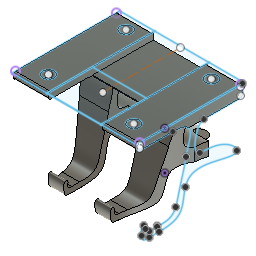
back-long (Autodesk Fusion 360 design; units mm, degrees)
Autodesk Fusion 360 part; units mm, degrees
sketch "Skizze1" plane through (0, 0, 0) normal (1, 0, 0) x (0, 1, 0)
  line L0 (-6.5006, 9.9908) -> (19.5, 9.9908)
  line L1 (20, 9.4908) -> (20, 8.1908)
  line L2 (-7.0006, 8.7446) -> (-7.0006, 9.4908)
  line L3 (-6.5006, 8.2446) -> (2, 8.2446)
  line L4 (10.0033, 7.0396) -> (19.4979, 7)
  line L5 (20, 7.5) -> (20, 8.1908)
  arc A0 (-6.5006, 9.9908) -> (-7.0006, 9.4908) centre (-6.5006, 9.4908) ccw
  arc A1 (-7.0006, 8.7446) -> (-6.5006, 8.2446) centre (-6.5006, 8.7446) ccw
  arc A2 (20, 9.4908) -> (19.5, 9.9908) centre (19.5, 9.4908) ccw
  arc A3 (19.4979, 7) -> (20, 7.5) centre (19.5, 7.5) ccw
  line L6 (-2, -11) -> (-2, -10.8002)
  spline S0 degree 5 poles (5.4564, 0.8875) (5.3855, 0.5136) (5.2329, -0.2254) (4.971, -1.3069) (4.5724, -2.7088) (4.0604, -4.4438) (3.5996, -6.1979) (3.1763, -7.9202) (2.7188, -9.497) (1.8719, -10.5223) (0.6223, -10.9522) (-0.5021, -11.0045) (-1.2907, -11.0008) (-1.7711, -11) (-2, -11) knots 0 0 0 0 0 0 0.1 0.2 0.3 0.4 0.5 0.6 0.7 0.8 0.9 1 1 1 1 1 1
  line L7 (-1, -11) -> (-3, -11)
  line L8 (5.6749, 2.0411) -> (5.2379, -0.266)
  spline S1 degree 5 poles (2, 8.2446) (2.8977, 8.2305) (4.4395, 8.0987) (5.9921, 7.5904) (6.778, 6.3951) (6.5221, 4.4543) (5.9835, 2.8697) (5.6586, 1.8097) (5.5121, 1.1818) (5.4564, 0.8875) knots 0 0 0 0 0 0 0.2 0.4 0.6 0.8 1 1 1 1 1 1
  line L9 (1.6903, 8.2495) -> (2.3097, 8.2397)
  line L10 (3.1911, -8.044) -> (2.3942, -9.956)
  line L11 (-1.4778, -12.3862) -> (-4, -12.3862)
  line L12 (-2, -11) -> (-4, -11)
  spline S2 degree 5 poles (-4, -12.3862) (-4.1637, -12.3825) (-4.4687, -12.3751) (-4.8588, -12.364) (-5.2518, -12.336) (-5.5755, -12.2143) (-5.7856, -11.9369) (-5.929, -11.4713) (-6.0363, -10.8339) (-6.0945, -10.1719) (-6.0772, -9.6063) (-5.9643, -9.2033) (-5.7546, -8.9907) (-5.4704, -8.9625) (-5.1907, -9.0678) (-5.0099, -9.2564) (-4.9465, -9.5244) (-4.9801, -9.8639) (-5.0384, -10.2433) (-5.0135, -10.5787) (-4.8541, -10.8326) (-4.5967, -10.9534) (-4.3278, -10.9955) (-4.1149, -11.0021) (-4, -11) knots 0 0 0 0 0 0 0.05 0.1 0.15 0.2 0.25 0.3 0.35 0.4 0.45 0.5 0.55 0.6 0.65 0.7 0.75 0.8 0.85 0.9 0.95 1 1 1 1 1 1
  line L13 (-3.0067, -12.4087) -> (-4.9933, -12.3637)
  line L14 (-5.782, -8.9412) -> (-5.1061, -9.0588)
  line L15 (-4.9315, -9.3688) -> (-5.0685, -10.6312)
  spline S3 degree 5 poles (-1.4778, -12.3862) (-0.8155, -12.3824) (0.4148, -12.3369) (1.9774, -12.1542) (3.4957, -11.6229) (4.4942, -10.2077) (4.8939, -8.0285) (5.1389, -5.3096) (6.4672, -3.4256) (9.3305, -3.0948) (13.0319, -3.8228) (16.5001, -4.7482) (18.6604, -4.9823) (18.8379, -4.0148) (17.5015, -2.4676) (15.2406, -1.0314) (12.6174, -0.2148) (10.1815, -0.0512) (8.3782, -0.213) (7.5748, 1.0515) (7.7465, 3.7291) (8.456, 5.8911) (9.1756, 6.8309) (9.7171, 7.0396) (10.0033, 7.0396) knots 0 0 0 0 0 0 0.05 0.1 0.15 0.2 0.25 0.3 0.35 0.4 0.45 0.5 0.55 0.6 0.65 0.7 0.75 0.8 0.85 0.9 0.95 1 1 1 1 1 1
  line L16 (-5.5492, -12.4096) -> (2.5937, -12.3628)
  line L17 (18.4871, -5.1308) -> (18.6154, -3.4332)
  line L18 (4.5138, -8.2258) -> (6.0937, -3.3604)
  line L19 (8.3709, 7.0396) -> (11.6358, 7.0396)
  line L20 (10.8658, -0.437) -> (7.1342, 0.437)
  line L21 (-5.8826, -11.7779) -> (-6.1174, -10.2221)
  point P0 (20, 9.9908)
  point P1 (2.7926, -9)
  point P2 (-6, -11)
  point P3 (-5.444, -9)
  point P4 (-5, -10)
  point P5 (5.3038, -5.7931)
  point P6 (18.5512, -4.282)
  point P7 (9, 0)
  dimension "d12" = 0.5
  constraint horizontal L0
  constraint perpendicular L0 L1
  constraint perpendicular L0 L2
  constraint perpendicular L2 L3
  constraint tangent L0 A0
  constraint tangent L2 A0
  constraint tangent L2 A1
  constraint tangent L3 A1
  constraint equal A0 A1
  constraint coincident P0 L0
  constraint coincident P0 L1
  constraint tangent L0 A2
  constraint tangent L1 A2
  constraint equal A0 A2
  constraint tangent L4 A3
  constraint tangent L5 A3
  constraint equal A0 A3
  constraint midpoint L8 S0.start
  constraint midpoint L3.end L9
  constraint midpoint P1 L10
  constraint midpoint L7 L6.start
  constraint midpoint L11.end L13
  constraint midpoint P3 L14
  constraint midpoint P4 L15
  constraint midpoint L11.start L16
  constraint midpoint P6 L17
  constraint midpoint P5 L18
  constraint midpoint L4.start L19
  constraint parallel L0 L19
  constraint midpoint P7 L20
  constraint midpoint P2 L21
  measures "d12" radius of A0
extrude "Extrusion1" add sketch "Skizze1" against normal blind 32 contours L0 L1 L2 L3 L4 L5 A0 A1 A2 A3 S0 L7 S1 L11 L12 S2 S3 makes body 1
sketch "Skizze2" plane through (0, 0, 9.9908) normal (0, 0, 1) x (-1, 0, 0)
  line L0 (0, 6.5006) -> (0, -19.5)
  line L1 (32, -19.5) -> (32, 6.5006)
  line L2 (16, 0) -> (16, -20) construction
  line L3 (0, -20.4) -> (0, 0)
  circle A0 centre (27, -17) radius 1.5
  circle A1 centre (5, -17) radius 1.5
  line L4 (32, -20.3851) -> (23, -20.3851)
  line L5 (23, -20.3851) -> (23, 7.4)
  line L6 (23, 7.4) -> (32, 7.4)
  line L7 (32, 7.4) -> (32, -20.3851)
  line L8 (0, -20.4) -> (9, -20.4)
  line L9 (9, -20.4) -> (9, 7.4031)
  line L10 (9, 7.4031) -> (0, 7.4031)
  line L11 (0, 7.4031) -> (0, -20.4)
  line L12 (23, -20.3851) -> (9, -20.3851)
  line L13 (9, -20.3851) -> (9, 7.4031)
  line L14 (9, 7.4031) -> (23, 7.4031)
  line L15 (23, 7.4031) -> (23, -20.3851)
  circle A2 centre (27, 3) radius 1.5
  circle A3 centre (5, 3) radius 1.5
  line L16 (23, 7.4) -> (9, 7.4)
  line L17 (9, 7.4) -> (9, -4.3434)
  line L18 (9, -4.3434) -> (23, -4.3434)
  line L19 (23, -4.3434) -> (23, 7.4)
  dimension "d6" = 3
  dimension "d7" = 3
  dimension "d23" = 3
  dimension "d24" = 3
  constraint coincident L3.end origin
  constraint horizontal L4
  constraint vertical L5
  constraint horizontal L6
  constraint vertical L7
  constraint horizontal L8
  constraint horizontal L10
  constraint vertical L11
  constraint horizontal L12
  constraint vertical L13
  constraint horizontal L14
  constraint vertical L15
  constraint horizontal L16
  constraint vertical L17
  constraint horizontal L18
  constraint vertical L19
  constraint coincident L9 L17.end
  constraint coincident L13 L17.end
  measures "d6" diameter of A0
  measures "d7" diameter of A1
  measures "d23" diameter of A2
  measures "d24" diameter of A3
extrude "Extrusion3" cut sketch "Skizze2" against normal blind 3 contours A0 | A1 bodies 1
sketch "Skizze3" plane through (0, 0, 0) normal (0, 0, 1) x (1, 0, 0)
  spline S0 degree 5 poles (0, 19.4997, -9.5) (0, 17.9511, -9.5) (-0.1634, 15.1033, -9.5) (-0.898, 11.5792, -9.5) (-2.6639, 8.0813, -9.5) (-5.3361, 4.4186, -9.5) (-7.102, 0.9208, -9.5) (-7.8366, -2.6034, -9.5) (-8, -5.4513, -9.5) (-8, -7, -9.5) knots 0 0 0 0 0 0 0.2 0.4 0.6 0.8 1 1 1 1 1 1
  line L0 (0, 21.4996, -9.5) -> (0, 17.4998, -9.5)
  line L1 (-8, -5, -9.5) -> (-8, -9, -9.5)
  line L2 (-16, 20, -9.5) -> (-16, -2, -9.5) construction
  line L3 (-12, 10.5, -9.5) -> (-20, 10.5, -9.5)
  line L4 (-20, 10.5, -9.5) -> (-20, -7, -9.5)
  line L5 (-20, -7, -9.5) -> (-12, -7, -9.5)
  line L6 (-12, -7, -9.5) -> (-12, 10.5, -9.5)
  line L7 (-8, -7, -9.5) -> (0, -7, -9.5)
  line L8 (0, -7, -9.5) -> (0, 19.4997, -9.5)
  line L9 (0, 15, -9.5) -> (0, 19.5, -9.5)
  line L10 (-1.1962, 20.6962, -9.5) -> (-5.8038, 20.6962, -9.5)
  line L11 (-7, 19.5, -9.5) -> (-7, 15, -9.5)
  arc A0 through (-7, 15, -9.5) (-6.5071, 13.81, -9.5) (-5.3171, 13.3171, -9.5)
  arc A1 through (-5.8038, 20.6962, -9.5) (-6.6496, 20.3458, -9.5) (-7, 19.5, -9.5)
  arc A2 through (0, 19.5, -9.5) (-0.3504, 20.3458, -9.5) (-1.1962, 20.6962, -9.5)
  line L12 (-5.3171, 13.3171, -9.5) -> (-2, 13.3171, -9.5)
  line L13 (-2, 13.3171, -9.5) -> (-2, 9.7247, -9.5)
  spline S1 degree 5 poles (0, 19.4997, -9.5) (0, 17.9511, -9.5) (-0.1634, 15.1033, -9.5) (-0.898, 11.5792, -9.5) (-2.6639, 8.0813, -9.5) (-5.3361, 4.4186, -9.5) (-7.102, 0.9208, -9.5) (-7.8366, -2.6034, -9.5) (-8, -5.4513, -9.5) (-8, -7, -9.5) knots 0 0 0 0 0 0 0.2 0.4 0.6 0.8 1 1 1 1 1 1
  line L14 (0, 21.4996, -9.5) -> (0, 17.4998, -9.5)
  line L15 (-8, -5, -9.5) -> (-8, -9, -9.5)
extrude "Extrusion5" cut sketch "Skizze2" against normal blind 1.8 contours L9 L13 L14 L15 L16 | L5 L9 L13 L15 L16 L17 L18 L19 | L5 L9 L12 L13 L15 L18 bodies 1
extrude "Extrusion7" cut sketch "Skizze3" along normal blind 16 and the other way blind 3 contours L3 L4 L5 L6 in plane through (0, 0, -9.5) normal (0, 0, 1) bodies 1
extrude "Extrusion8" cut sketch "Skizze2" against normal blind 3 contours A2 | A3 bodies 1
extrude "Extrusion13" add sketch "Skizze3" along normal blind 16.5 and the other way blind 3 separate body contours S0 L0 L7 L8 L9 S1 L14 | S0 L10 L11 A0 A1 A2 L12 L13 S1 in plane through (0, 0, -9.5) normal (0, 0, 1) makes body 2
mirror "Spiegeln1" about plane through (0, 19.4997, -9.5) normal (1, 0, 0) of bodies 2 makes body 3
move_body "Verschieben1" bodies 3 to x (1, 0, 0) y (0, 1, 0) z (0, 0, 1) at (-32, 0, 0)
combine "Kombinieren1" operation cut target body 1 tool bodies 3 2
extrude "Extrusion14" cut sketch "Skizze2" against normal blind 4 contours L5 L9 L13 L15 L16 L17 L18 L19 bodies 1
